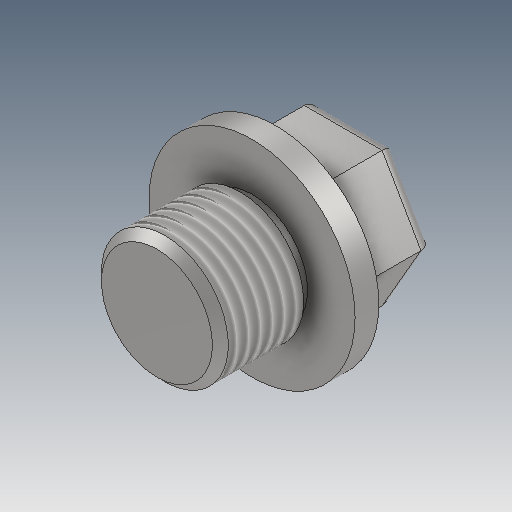
# Autodesk Inventor part: 排油孔螺塞
Saved by Autodesk Inventor 2025 (Build 290162000, 162)
## iProperties
Created: 2025-03-14
Part Number: 排油孔螺塞
Material: 钢，软
Document SubType Name: Modeling
Designer: ASUS
Density: 7.85 g/cm^3
Appearance: 不锈钢 - 拉丝
Author: ASUS
Autodesk Inventor part; units mm, degrees
ref_plane "YZ Plane" through (0, 0, 0) normal (1, 0, 0) x (0, 1, 0)
ref_plane "XZ Plane" through (0, 0, 0) normal (0, 1, 0) x (-1, 0, 0)
ref_plane "XY Plane" through (0, 0, 0) normal (0, 0, 1) x (1, 0, 0)
sketch "草图1" plane through (0, 0, 0) normal (0, 1, 0) x (-1, 0, 0)
  line L0 (0, 0) -> (13, 0)
  line L1 (13, 0) -> (13, 3)
  line L2 (13, 3) -> (7, 3)
  line L3 (7, 3) -> (7, 4.5)
  line L4 (7, 4.5) -> (8, 4.5)
  line L5 (8, 4.5) -> (8, 15)
  line L6 (8, 15) -> (0, 15)
  line L7 (0, 15) -> (0, 0)
  dimension "d0" = 13
  dimension "d2" = 3
  dimension "d3" = 1.5
  dimension "d4" = 1
  dimension "d5" = 8
  dimension "d6" = 12
  constraints: 16 end point, 7 perpendicular, 1 horizontal
  measures "d0" distance of L0.start L0.end
  measures "d2" distance of L0.end L1.end
  measures "d3" distance of L2.end L3.end
  measures "d4" distance of L3.end L4.end
  measures "d5" distance between parallel lines of L7 L5
  measures "d6" distance between parallel lines of L2 L6
revolve "旋转1" add sketch "草图1" angle 360 about axis through (0, 0, 15) along (0, 0, -1)
chamfer "倒角1" distance 1 angle 45 1 edges at (8, 0, 15)
thread "螺纹1" size "M16x1.5" class "6g" standard "GB Metric profile" length 20
sketch "草图2" plane through (0, 0, 0) normal (0, 0, -1) x (-1, 0, 0)
  circle A0 centre (0, 0) radius 8 projected
  line L0 (9.815, 0) -> (4.9075, -8.5)
  line L1 (4.9075, -8.5) -> (-4.9075, -8.5)
  line L2 (-4.9075, -8.5) -> (-9.815, 0)
  line L3 (-9.815, 0) -> (-4.9075, 8.5)
  line L4 (-4.9075, 8.5) -> (4.9075, 8.5)
  line L5 (4.9075, 8.5) -> (9.815, 0)
  point P0 (0, 0)
  dimension "d13" = 17
  constraints: 12 end point, 1 coincident, 13 other
  measures "d13" distance between parallel lines of L1 L4
extrude "拉伸1" add sketch "草图2" along normal blind 10 contours A0 | L0 L1 L2 L3 L4 L5
fillet "圆角1" radius 1.5 6 edges at (0, -8.5, -10) (7.3612, -4.25, -10) (7.3612, 4.25, -10) (0, 8.5, -10) (-7.3612, 4.25, -10) (-7.3612, -4.25, -10)
equation "\"d0\" = 0.5 * D0"
equation "\"d2\" = a"
equation "\"d5\" = 0.5 * d"
equation "\"d6\" = l_"
equation "\"d\" = 16"
equation "\"D0\" = 26"
equation "\"L\" = 23"
equation "\"l_\" = 12"
equation "\"a\" = 3"
equation "\"D\" = 19.6"
equation "\"S_\" = 17"
equation "\"D1\" = 16.2"
equation "\"d1\" = 17"
equation "\"H_\" = 2"
